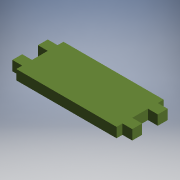
# Autodesk Inventor part: Middle_leg_c
Saved by Autodesk Inventor 2017 (Build 210142000, 142)
## iProperties
Part Number: Middle_leg_c
Material: Generic
Document SubType Name: Modeling
Designer: Alexander Miller
Appearance: Olive Green
Author: Alexander Miller
Autodesk Inventor part; units mm, degrees
ref_plane "YZ Plane" through (0, 0, 0) normal (1, 0, 0) x (0, 1, 0)
ref_plane "XZ Plane" through (0, 0, 0) normal (0, 1, 0) x (-1, 0, 0)
ref_plane "XY Plane" through (0, 0, 0) normal (0, 0, 1) x (1, 0, 0)
sketch "Sketch1" plane through (0, 0, 0) normal (0, 1, 0) x (-1, 0, 0)
  line L0 (25.5, 12) -> (-25.5, 12)
  line L1 (-25.5, 12) -> (-25.5, -12)
  line L2 (-25.5, -12) -> (25.5, -12)
  line L3 (25.5, -12) -> (25.5, 12)
  line L4 (25.5, 9) -> (30.5, 9)
  line L5 (30.5, 9) -> (30.5, 4)
  line L6 (30.5, 4) -> (25.5, 4)
  line L7 (25.5, 4) -> (25.5, 9)
  line L8 (41.3, 0) -> (-41.3, 0) projected
  line L9 (25.5, -9) -> (30.5, -9)
  line L10 (30.5, -9) -> (30.5, -4)
  line L11 (30.5, -4) -> (25.5, -4)
  line L12 (25.5, -4) -> (25.5, -9)
  line L13 (0, -16.8) -> (0, 16.8) projected
  line L14 (-25.5, 9) -> (-30.5, 9)
  line L15 (-30.5, 9) -> (-30.5, 4)
  line L16 (-30.5, 4) -> (-25.5, 4)
  line L17 (-25.5, 4) -> (-25.5, 9)
  line L18 (-30.5, -9) -> (-30.5, -4)
  line L19 (-25.5, -9) -> (-30.5, -9)
  line L20 (-30.5, -4) -> (-25.5, -4)
  line L21 (-25.5, -4) -> (-25.5, -9)
  point P0 (0, 0)
  point P1 (25.5, 0)
  point P2 (0, 12)
  point P3 (-25.5, 0)
  dimension "d0" = 5
  dimension "d1" = 5
  dimension "d2" = 4
  dimension "d3" = 24
  dimension "d4" = 51
  constraints: 40 end point, 13 symmetric about line, 4 parallel, 2 horizontal, 2 midpoint, 2 perpendicular, 1 horizontal alignment, 1 point on line, 1 vertical alignment
  measures "d0" distance of L4.end L5.end
  measures "d1" distance of L4.start L4.end
  measures "d2" distance between parallel lines of L8 L6
  measures "d3" distance of L2.end L0.start
  measures "d4" distance between parallel lines of L1 L3
extrude "Extrusion1" add sketch "Sketch1" along normal blind 5
equation "\"d0\" = b_mat_thickness"
equation "\"d1\" = b_mat_thickness"
equation "\"d2\" = 0.8 * b_mat_thickness"
equation "\"d3\" = sa_diameter"
equation "\"d4\" = b_mat_thickness + s_shaft_height + s_height + sa_thickness"
equation "\"d5\" = b_mat_thickness"
equation "\"b_mat_thickness\" = 5"
equation "\"sa_diameter\" = 24"
equation "\"s_shaft_height\" = 6"
equation "\"s_height\" = 38"
equation "\"sa_thickness\" = 2"
body "Solid1"
